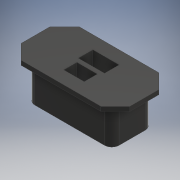
# Autodesk Inventor part: BA28
Saved by Autodesk Inventor 2017 (Build 210142000, 142)
## iProperties
Created: 2019-06-14
Part Number: BA28
Material: ABS Plastic
Document SubType Name: Modeling
Designer: Dell
Density: 1.06 g/cm^3
Appearance: Smooth - Black
Author: Dell
Autodesk Inventor part; units mm, degrees
ref_plane "YZ Plane" through (0, 0, 0) normal (1, 0, 0) x (0, 1, 0)
ref_plane "XZ Plane" through (0, 0, 0) normal (0, 1, 0) x (-1, 0, 0)
ref_plane "XY Plane" through (0, 0, 0) normal (0, 0, 1) x (1, 0, 0)
sketch "Sketch1" plane through (0, 0, 0) normal (0, 0, 1) x (1, 0, 0)
  line L0 (0, 0) -> (58, 0)
  line L1 (58, 0) -> (58, 28)
  line L2 (58, 28) -> (0, 28)
  line L3 (0, 28) -> (0, 0)
  line L4 (22, 12) -> (36, 12)
  line L5 (36, 12) -> (36, 3)
  line L6 (36, 3) -> (22, 3)
  line L7 (22, 3) -> (22, 12)
  line L8 (20, 25) -> (38, 25)
  line L9 (38, 25) -> (38, 15)
  line L10 (38, 15) -> (20, 15)
  line L11 (20, 15) -> (20, 25)
  line L12 (29, 25) -> (29, 3) construction
  point P0 (29, 28)
  point P1 (29, 12)
  point P2 (29, 14)
  point P3 (0, 14)
  dimension "d0" = 14
  dimension "d1" = 9
  dimension "d2" = 28
  dimension "d3" = 58
  dimension "d4" = 18
  dimension "d5" = 10
  dimension "d6" = 3
  constraints: 26 end point, 6 midpoint, 6 parallel, 3 horizontal, 3 perpendicular, 2 vertical alignment, 1 horizontal alignment
  measures "d0" distance of L5.end L6.end
  measures "d1" distance of L4.end L5.end
  measures "d2" distance of L2.end L0.start
  measures "d3" distance of L0.start L0.end
  measures "d4" distance of L9.end L10.end
  measures "d5" distance of L8.end L9.end
  measures "d6" distance between parallel lines of L10 L4
extrude "Extrusion1" add sketch "Sketch1" along normal blind 25
fillet "Fillet1" radius 5 4 edges at (0, 28, 12.5) (0, 0, 12.5) (58, 0, 12.5) (58, 28, 12.5)
sketch "Sketch2" plane through (0, 0, 25) normal (0, 0, 1) x (1, 0, 0)
  arc A0 (58, 23) -> (53, 28) centre (53, 23) ccw projected
  line L0 (53, 28) -> (5, 28) projected
  arc A1 (5, 28) -> (0, 23) centre (5, 23) ccw projected
  line L1 (0, 23) -> (0, 5) projected
  arc A2 (0, 5) -> (5, 0) centre (5, 5) ccw projected
  line L2 (5, 0) -> (53, 0) projected
  arc A3 (53, 0) -> (58, 5) centre (53, 5) ccw projected
  line L3 (58, 5) -> (58, 23) projected
  line L4 (38, 25) -> (38, 15) projected
  line L5 (38, 15) -> (20, 15) projected
  line L6 (20, 15) -> (20, 25) projected
  line L7 (20, 25) -> (38, 25) projected
  line L8 (36, 12) -> (36, 3) projected
  line L9 (36, 3) -> (22, 3) projected
  line L10 (22, 3) -> (22, 12) projected
  line L11 (22, 12) -> (36, 12) projected
  line L12 (-8.5, 34) -> (66.5, 34)
  line L13 (66.5, 34) -> (66.5, -6)
  line L14 (66.5, -6) -> (-8.5, -6)
  line L15 (-8.5, -6) -> (-8.5, 34)
  point P0 (29, 34)
  point P1 (29, 28)
  point P2 (0, 14)
  point P3 (-8.5, 14)
  dimension "d11" = 40
  dimension "d12" = 75
  constraints: 8 end point, 4 midpoint, 2 parallel, 1 horizontal, 1 horizontal alignment, 1 perpendicular, 1 vertical alignment
  measures "d11" distance of L14.end L12.start
  measures "d12" distance of L12.start L12.end
extrude "Extrusion2" add sketch "Sketch2" along normal blind 3 contours L3 A3 L2 A2 L1 A1 L0 A0 | L12 L13 L14 L15
chamfer "Chamfer1" distance 10 angle 45 4 edges at (-8.5, 34, 26.5) (-8.5, -6, 26.5) (66.5, 34, 26.5) (66.5, -6, 26.5)
body "Solid1"
